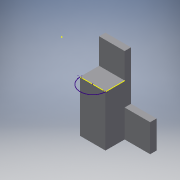
# Autodesk Inventor part: Part43
Saved by Autodesk Inventor 2016 (Build 200138000, 138)
## iProperties
Created: 2016-01-27
Part Number: Part43
Material: Generic
Document SubType Name: Modeling
Designer: seve
Density: 1 g/cm^3
Appearance: Default
Author: seve
Autodesk Inventor part; units mm, degrees
ref_plane "YZ Plane" through (0, 0, 0) normal (1, 0, 0) x (0, 1, 0)
ref_plane "XZ Plane" through (0, 0, 0) normal (0, 1, 0) x (-1, 0, 0)
ref_plane "XY Plane" through (0, 0, 0) normal (0, 0, 1) x (1, 0, 0)
sketch "Sketch1" plane through (0, 0, 0) normal (0, 0, 1) x (1, 0, 0)
  line L0 (17.229, 11.486) -> (10.879, 11.486)
  line L1 (10.879, 11.486) -> (10.879, -1.214)
  line L2 (10.879, -1.214) -> (17.229, -1.214)
  line L3 (17.229, -1.214) -> (17.229, 11.486)
  point P0 (0, 0)
  dimension "d0" = 6.35
  dimension "d1" = 12.7
  constraints: 8 end point, 2 parallel, 1 horizontal, 1 perpendicular
  measures "d0" distance of L1.end L2.end
  measures "d1" distance of L2.end L0.start
extrude "Extrusion1" add sketch "Sketch1" along normal blind 6.35
sketch "Sketch2" plane through (10.879, 11.486, 0) normal (0, 1, 0) x (1, 0, 0)
  line L0 (6.35, 0) -> (6.35, -6.35) projected
  line L1 (6.35, 0) -> (0, 0) projected
  line L2 (6.35, -1.5875) -> (0, -1.5875)
  line L3 (0, -1.5875) -> (0, 0)
  line L4 (0, 0) -> (6.35, 0)
  line L5 (6.35, 0) -> (6.35, -1.5875)
  point P0 (-10.879, 0)
  dimension "d6" = 1.5875
  constraints: 8 end point, 2 parallel, 1 horizontal, 1 perpendicular, 1 point on line
  measures "d6" distance between parallel lines of L1 L2
extrude "Extrusion2" add sketch "Sketch2" along normal blind 6.35
sketch "Sketch3" plane through (17.229, -1.214, 6.35) normal (1, 0, 0) x (0, 0, -1)
  line L0 (6.35, 0) -> (0, 0) projected
  line L1 (6.35, 0) -> (6.35, 19.05) projected
  line L2 (4.7625, 0) -> (6.35, 0)
  line L3 (6.35, 0) -> (6.35, 6.8907)
  line L4 (6.35, 6.8907) -> (4.7625, 6.8907)
  line L5 (4.7625, 6.8907) -> (4.7625, 0)
  point P0 (6.35, 1.214)
  dimension "d7" = 1.5875
  constraints: 8 end point, 2 parallel, 2 point on line, 1 horizontal, 1 perpendicular
  measures "d7" distance of L3.end L4.end
extrude "Extrusion3" add sketch "Sketch3" along normal blind 6.35
sketch "Sketch5" plane through (10.879, 11.486, 1.5875) normal (0, 1, 0) x (1, 0, 0)
  line L0 (0, 0) -> (0, -4.7625) projected
  line L1 (6.35, 0) -> (6.35, -4.7625) projected
  point P0 (-10.879, 1.5875)
body "Solid1"
